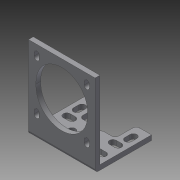
# Autodesk Inventor part: holder
Saved by Autodesk Inventor 2015 (Build 190159000, 159)
## iProperties
Created: 2017-03-08
Part Number: holder
Material: Generic
Document SubType Name: Modeling
Designer: Guy
Density: 1 g/cm^3
Appearance: Default
Mass: 5.81575 g
Surface Area: 56.9676 cm^2
Volume: 5.81575 cm^3
Author: Guy
Autodesk Inventor part; units mm, degrees
ref_plane "YZ Plane" through (0, 0, 0) normal (1, 0, 0) x (0, 1, 0)
ref_plane "XZ Plane" through (0, 0, 0) normal (0, 1, 0) x (-1, 0, 0)
ref_plane "XY Plane" through (0, 0, 0) normal (0, 0, 1) x (1, 0, 0)
sketch "Sketch1" plane through (0, 0, 0) normal (0, 0, 1) x (1, 0, 0)
  line L0 (0, 0) -> (41.3, 0)
  line L1 (41.3, 0) -> (41.3, 35)
  line L2 (41.3, 35) -> (0, 35)
  line L3 (0, 35) -> (0, 0)
  dimension "d0" = 41.3
  dimension "d1" = 35
  constraints: 8 end point, 2 parallel, 1 horizontal, 1 perpendicular
  measures "d0" distance of L1.end L2.end
  measures "d1" distance of L0.end L1.end
extrude "Extrusion1" add sketch "Sketch1" along normal blind 3
sketch "Sketch2" plane through (0, 0, 3) normal (0, 0, 1) x (1, 0, 0)
  line L0 (0, 0) -> (41.3, 0)
  line L1 (41.3, 0) -> (41.3, 3)
  line L2 (41.3, 3) -> (0, 3)
  line L3 (0, 3) -> (0, 0)
  line L4 (41.3, 0) -> (41.3, 35) projected
  dimension "d4" = 3
  constraints: 8 end point, 2 parallel, 1 horizontal, 1 perpendicular, 1 point on line
  measures "d4" distance between parallel lines of L0 L2
extrude "Extrusion2" add sketch "Sketch2" along normal blind 48
fillet "Fillet1" radius 2 1 edges at (20.65, 0, 0)
sketch "Sketch3" plane through (0, 0, 3) normal (0, 0, 1) x (1, 0, 0)
  arc A0 (4.75, 11.65) -> (4.75, 7.35) centre (4.75, 9.5) ccw
  arc A1 (7.95, 7.35) -> (7.95, 11.65) centre (7.95, 9.5) ccw
  arc A2 (4.75, 21.15) -> (4.75, 16.85) centre (4.75, 19) ccw
  arc A3 (7.95, 16.85) -> (7.95, 21.15) centre (7.95, 19) ccw
  arc A4 (2.6, 25.3) -> (6.9, 25.3) centre (4.75, 25.3) ccw
  arc A5 (6.9, 28.5) -> (2.6, 28.5) centre (4.75, 28.5) ccw
  line L0 (2.6, 25.3) -> (2.6, 28.5)
  line L1 (4.75, 7.35) -> (7.95, 7.35)
  line L2 (4.75, 11.65) -> (7.95, 11.65)
  line L3 (4.75, 16.85) -> (7.95, 16.85)
  line L4 (4.75, 21.15) -> (7.95, 21.15)
  line L5 (6.9, 25.3) -> (6.9, 28.5)
  line L6 (41.3, 3) -> (0, 3) projected
  line L7 (0, 35) -> (0, 3) projected
  line L8 (0, 0) -> (41.3, 0) projected
  line L9 (20.65, 38.1928) -> (20.65, -3.6138)
  arc A6 (12.15, 9.5) -> (16.45, 9.5) centre (14.3, 9.5) ccw
  arc A7 (16.45, 12.7) -> (12.15, 12.7) centre (14.3, 12.7) ccw
  circle A8 centre (20.65, 9.5) radius 2.15
  line L10 (12.15, 9.5) -> (12.15, 12.7)
  line L11 (16.45, 9.5) -> (16.45, 12.7)
  arc A9 (36.55, 7.35) -> (36.55, 11.65) centre (36.55, 9.5) ccw
  arc A10 (33.35, 11.65) -> (33.35, 7.35) centre (33.35, 9.5) ccw
  arc A11 (36.55, 16.85) -> (36.55, 21.15) centre (36.55, 19) ccw
  arc A12 (33.35, 21.15) -> (33.35, 16.85) centre (33.35, 19) ccw
  arc A13 (34.4, 25.3) -> (38.7, 25.3) centre (36.55, 25.3) ccw
  arc A14 (38.7, 28.5) -> (34.4, 28.5) centre (36.55, 28.5) ccw
  line L12 (38.7, 25.3) -> (38.7, 28.5)
  line L13 (36.55, 7.35) -> (33.35, 7.35)
  line L14 (36.55, 11.65) -> (33.35, 11.65)
  line L15 (36.55, 16.85) -> (33.35, 16.85)
  line L16 (36.55, 21.15) -> (33.35, 21.15)
  line L17 (34.4, 25.3) -> (34.4, 28.5)
  arc A15 (24.85, 9.5) -> (29.15, 9.5) centre (27, 9.5) ccw
  arc A16 (29.15, 12.7) -> (24.85, 12.7) centre (27, 12.7) ccw
  line L18 (29.15, 9.5) -> (29.15, 12.7)
  line L19 (24.85, 9.5) -> (24.85, 12.7)
  dimension "d8" = 4.3
  dimension "d9" = 4.3
  dimension "d10" = 4.3
  dimension "d11" = 9.5
  dimension "d12" = 9.5
  dimension "d13" = 9.5
  dimension "d14" = 3.2
  dimension "d15" = 20.65
  dimension "d16" = 15.9
  dimension "d17" = 15.9
  dimension "d18" = 15.9
  dimension "d19" = 3.2
  dimension "d20" = 3.2
  dimension "d21" = 4.3
  dimension "d22" = 9.5
  dimension "d23" = 3.2
  dimension "d24" = 4.3
  dimension "d25" = 9.5
  dimension "d26" = 6.35
  constraints: 34 end point, 32 point on circle, 24 symmetric about line, 17 centre point, 16 tangent, 5 parallel, 5 vertical, 1 point on line, 8 other
  measures "d8" diameter of A0
  measures "d9" diameter of A2
  measures "d10" diameter of A4
  measures "d11" distance from line of L8 A0.centre
  measures "d12" distance of A0.centre A2.centre
  measures "d13" distance of A2.centre A5.centre
  measures "d14" distance of A4.centre A5.centre
  measures "d15" distance between parallel lines of L9 L7
  measures "d16" distance from line of L9 A5.centre
  measures "d17" distance from line of L9 A2.centre
  measures "d18" distance from line of L9 A0.centre
  measures "d19" distance of A1.centre A0.centre
  measures "d20" distance of A3.centre A2.centre
  measures "d21" diameter of A8
  measures "d22" distance from line of L8 A8.centre
  measures "d23" distance of A6.centre A7.centre
  measures "d24" diameter of A7
  measures "d25" distance from line of L8 A6.centre
  measures "d26" distance from line of L9 A6.centre
extrude "Extrusion3" cut sketch "Sketch3" against normal up to next
sketch "Sketch4" plane through (0, 0, 3) normal (0, 0, 1) x (1, 0, 0)
  arc A0 (36.55, 16.85) -> (36.55, 21.15) centre (36.55, 19) ccw projected
  line L0 (36.55, 16.85) -> (33.35, 16.85) projected
  arc A1 (33.35, 21.15) -> (33.35, 16.85) centre (33.35, 19) ccw projected
  line L1 (33.35, 21.15) -> (36.55, 21.15) projected
  arc A2 (24.85, 9.5) -> (29.15, 9.5) centre (27, 9.5) ccw projected
  line L2 (24.85, 9.5) -> (24.85, 12.7) projected
  arc A3 (29.15, 12.7) -> (24.85, 12.7) centre (27, 12.7) ccw projected
  line L3 (29.15, 12.7) -> (29.15, 9.5) projected
  arc A4 (7.95, 16.85) -> (7.95, 21.15) centre (7.95, 19) ccw projected
  line L4 (7.95, 16.85) -> (4.75, 16.85) projected
  arc A5 (4.75, 21.15) -> (4.75, 16.85) centre (4.75, 19) ccw projected
  line L5 (4.75, 21.15) -> (7.95, 21.15) projected
  arc A6 (2.6, 25.3) -> (6.9, 25.3) centre (4.75, 25.3) ccw projected
  line L6 (2.6, 25.3) -> (2.6, 28.5) projected
  arc A7 (6.9, 28.5) -> (2.6, 28.5) centre (4.75, 28.5) ccw projected
  line L7 (6.9, 28.5) -> (6.9, 25.3) projected
  circle A8 centre (20.65, 9.5) radius 2.15 projected
  arc A9 (7.95, 7.35) -> (7.95, 11.65) centre (7.95, 9.5) ccw projected
  line L8 (7.95, 7.35) -> (4.75, 7.35) projected
  arc A10 (4.75, 11.65) -> (4.75, 7.35) centre (4.75, 9.5) ccw projected
  line L9 (4.75, 11.65) -> (7.95, 11.65) projected
  arc A11 (12.15, 9.5) -> (16.45, 9.5) centre (14.3, 9.5) ccw projected
  line L10 (12.15, 9.5) -> (12.15, 12.7) projected
  arc A12 (16.45, 12.7) -> (12.15, 12.7) centre (14.3, 12.7) ccw projected
  line L11 (16.45, 12.7) -> (16.45, 9.5) projected
  arc A13 (36.55, 7.35) -> (36.55, 11.65) centre (36.55, 9.5) ccw projected
  line L12 (36.55, 7.35) -> (33.35, 7.35) projected
  arc A14 (33.35, 11.65) -> (33.35, 7.35) centre (33.35, 9.5) ccw projected
  line L13 (33.35, 11.65) -> (36.55, 11.65) projected
  arc A15 (38.7, 28.5) -> (34.4, 28.5) centre (36.55, 28.5) ccw projected
  line L14 (38.7, 28.5) -> (38.7, 25.3) projected
  arc A16 (34.4, 25.3) -> (38.7, 25.3) centre (36.55, 25.3) ccw projected
  line L15 (34.4, 25.3) -> (34.4, 28.5) projected
  line L16 (0, 3) -> (41.3, 3) projected
  line L17 (41.3, 3) -> (41.3, 35) projected
  line L18 (41.3, 35) -> (0, 35) projected
  line L19 (0, 35) -> (0, 3) projected
  line L20 (41.3, 35) -> (0, 35) projected
  line L21 (0, 35) -> (0, 3) projected
  line L22 (41.3, 3) -> (41.3, 35) projected
  line L23 (9.55, 35) -> (9.55, 22)
  line L24 (9.55, 22) -> (18.5, 22)
  line L25 (18.5, 22) -> (18.5, 16.85)
  line L26 (18.5, 16.85) -> (22.8, 16.85)
  line L27 (22.8, 16.85) -> (22.8, 22)
  line L28 (22.8, 22) -> (31.75, 22)
  line L29 (31.75, 22) -> (31.75, 35)
  circle A17 centre (20.65, 9.5) radius 2.15 projected
  arc A18 (7.95, 16.85) -> (7.95, 21.15) centre (7.95, 19) ccw projected
  line L30 (9.55, 35) -> (31.75, 35)
  point P0 (0, 0)
  dimension "d34" = 22.2
  dimension "d36" = 13
  dimension "d37" = 11.1
  constraints: 16 end point, 6 perpendicular, 4 point on line, 3 tangent, 1 collinear
  measures "d34" distance between parallel lines of L29 L23
  measures "d36" distance between parallel lines of L28 L20
  measures "d37" distance from line of A8.centre L23
extrude "Extrusion4" cut sketch "Sketch4" against normal up to next contours L18 L29 L28 L27 L26 L25 L24 L23
fillet "Fillet2" radius 2.15 8 edges at (18.5, 16.85, 1.5) (22.8, 16.85, 1.5) (22.8, 22, 1.5) (18.5, 22, 1.5) (9.55, 22, 1.5) (31.75, 22, 1.5) (9.55, 35, 1.5) (31.75, 35, 1.5)
sketch "Sketch5" plane through (0, 0, 51) normal (0, -1, 0) x (1, 0, 0)
  arc A0 (4.6813, -21.6) -> (36.6187, -21.6) centre (20.65, -22.6) ccw
  line L0 (41.3, -49) -> (41.3, 0) projected
  line L1 (0, -51) -> (41.3, -51) projected
  arc A1 (6.75, -5.1) -> (3.55, -5.1) centre (5.15, -5.1) ccw
  arc A2 (3.55, -7.1) -> (6.75, -7.1) centre (5.15, -7.1) ccw
  line L2 (3.55, -5.1) -> (3.55, -7.1)
  line L3 (6.75, -5.1) -> (6.75, -7.1)
  arc A3 (6.75, -36.1) -> (3.55, -36.1) centre (5.15, -36.1) ccw
  arc A4 (3.55, -38.1) -> (6.75, -38.1) centre (5.15, -38.1) ccw
  line L4 (3.55, -36.1) -> (3.55, -38.1)
  line L5 (6.75, -36.1) -> (6.75, -38.1)
  arc A5 (37.75, -5.1) -> (34.55, -5.1) centre (36.15, -5.1) ccw
  arc A6 (34.55, -7.1) -> (37.75, -7.1) centre (36.15, -7.1) ccw
  line L6 (34.55, -5.1) -> (34.55, -7.1)
  line L7 (37.75, -5.1) -> (37.75, -7.1)
  arc A7 (37.75, -36.1) -> (34.55, -36.1) centre (36.15, -36.1) ccw
  arc A8 (34.55, -38.1) -> (37.75, -38.1) centre (36.15, -38.1) ccw
  line L8 (34.55, -36.1) -> (34.55, -38.1)
  line L9 (37.75, -36.1) -> (37.75, -38.1)
  arc A9 (36.6187, -21.6) -> (4.6813, -21.6) centre (20.65, -20.6) ccw
  dimension "d41" = 32
  dimension "d42" = 20.65
  dimension "d43" = 28.4
  dimension "d44" = 3.2
  dimension "d45" = 3.2
  dimension "d46" = 2
  dimension "d47" = 3.2
  dimension "d48" = 3.2
  dimension "d49" = 2
  dimension "d50" = 3.2
  dimension "d51" = 3.2
  dimension "d52" = 2
  dimension "d53" = 3.2
  dimension "d54" = 3.2
  dimension "d55" = 2
  dimension "d56" = 15.5
  dimension "d57" = 15.5
  dimension "d58" = 15.5
  dimension "d59" = 15.5
  dimension "d60" = 14.9
  dimension "d61" = 14.9
  dimension "d62" = 31
  dimension "d63" = 31
  dimension "d64" = 32
  dimension "d65" = 2
  dimension "d66" = 20.65
  constraints: 20 point on circle, 16 end point, 16 tangent, 10 centre point, 4 vertical
  measures "d41" diameter of A0
  measures "d42" distance from line of A0.centre L0
  measures "d43" distance from line of L1 A0.centre
  measures "d44" diameter of A1
  measures "d45" diameter of A2
  measures "d46" distance of A2.centre A1.centre
  measures "d47" diameter of A3
  measures "d48" diameter of A4
  measures "d49" distance of A4.centre A3.centre
  measures "d50" diameter of A5
  measures "d51" diameter of A6
  measures "d52" distance of A6.centre A5.centre
  measures "d53" diameter of A7
  measures "d54" diameter of A8
  measures "d55" distance of A8.centre A7.centre
  measures "d56" horizontal distance of A4.centre A0.centre
  measures "d57" horizontal distance of A8.centre A0.centre
  measures "d58" horizontal distance of A0.centre A5.centre
  measures "d59" horizontal distance of A1.centre A0.centre
  measures "d60" distance from line of A3.centre L1
  measures "d61" distance from line of L1 A7.centre
  measures "d62" distance of A1.centre A3.centre
  measures "d63" distance of A5.centre A7.centre
  measures "d64" diameter of A9
  measures "d65" distance of A0.centre A9.centre
  measures "d66" distance from line of L0 A9.centre
extrude "Extrusion5" cut sketch "Sketch5" against normal up to next
body "Solid1"
